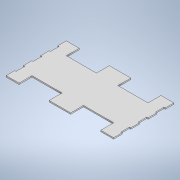
# Autodesk Inventor part: onderkant
Saved by Autodesk Inventor 2021 (Build 250183000, 183)
## iProperties
Created: 2022-02-01
Part Number: onderkant
Material: Generic
Document SubType Name: Modeling
Designer: ryan
Density: 1 g/cm^3
Appearance: Default
Author: ryan
Autodesk Inventor part; units mm, degrees
ref_plane "YZ Plane" through (0, 0, 0) normal (1, 0, 0) x (0, 1, 0)
ref_plane "XZ Plane" through (0, 0, 0) normal (0, 1, 0) x (-1, 0, 0)
ref_plane "XY Plane" through (0, 0, 0) normal (0, 0, 1) x (1, 0, 0)
sketch "Sketch1" plane through (0, 0, 0) normal (0, 1, 0) x (-1, 0, 0)
  line L0 (0, 0) -> (250, 0)
  line L1 (0, -140) -> (0, 0)
  line L2 (250, 0) -> (250, -70)
  line L3 (250, 0) -> (125, 0)
  line L4 (125, 0) -> (125, -70)
  line L5 (125, -70) -> (250, -70)
  line L6 (250, -70) -> (250, 0)
  line L7 (250, 0) -> (220, 0)
  line L8 (220, 0) -> (220, -30)
  line L9 (220, -30) -> (150, -30)
  line L10 (150, -30) -> (150, 0)
  line L11 (250, 0) -> (247, 0)
  line L12 (247, 0) -> (247, -20)
  line L13 (247, -20) -> (250, -20)
  line L14 (247, -20) -> (247, -70)
  line L15 (250, -20) -> (250, -40)
  line L16 (250, -40) -> (250, -60)
  line L17 (250, -60) -> (247, -60)
  line L18 (250, -40) -> (247, -40)
  dimension "d2" = 125
  dimension "d3" = 70
  dimension "d5" = 30
  dimension "d6" = 70
  dimension "d7" = 3
  dimension "d8" = 20
  dimension "d9" = 20
  dimension "d10" = 20
  constraints: 38 end point, 10 point on line, 6 perpendicular, 3 horizontal, 2 parallel, 1 vertical
  measures "d2" distance of L5.end L4.end
  measures "d3" distance of L4.end L3.end
  measures "d5" distance of L7.end L8.end
  measures "d6" distance of L8.end L9.end
  measures "d7" distance of L0.end L11.end
  measures "d8" distance of L11.end L12.end
  measures "d9" distance of L13.end L15.end
  measures "d10" distance of L15.end L16.end
extrude "Extrusion1" add sketch "Sketch1" along normal blind 3 contours L0 L10 L9 L8 L12 L14 L5 L4 | L0 L2 L13 L12 | L14 L18 L2 L17
mirror "Mirror1" about plane through (-125, 0, -70) normal (0, 0, -1) of "Extrusion1"
mirror "Mirror2" about plane through (-125, 0, 0) normal (1, 0, 0) of "Extrusion1", "Mirror1"
body "Solid1"
